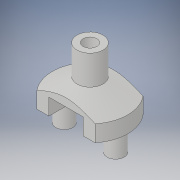
# Autodesk Inventor part: 1216.1001
Saved by Autodesk Inventor 2019.4 (Build 234330000, 330)
## iProperties
Created: 2019-11-11
Part Number: 1216.1001
Material: Generic
Document SubType Name: Modeling
Designer: phpgb
Density: 1 g/cm^3
Appearance: Default
Author: phpgb
Autodesk Inventor part; units mm, degrees
ref_plane "YZ Plane" through (0, 0, 0) normal (1, 0, 0) x (0, 1, 0)
ref_plane "XZ Plane" through (0, 0, 0) normal (0, 1, 0) x (-1, 0, 0)
ref_plane "XY Plane" through (0, 0, 0) normal (0, 0, 1) x (1, 0, 0)
sketch "Sketch1" plane through (0, 0, 0) normal (0, 1, 0) x (-1, 0, 0)
  line L0 (5.5, 3.5) -> (4.2426, 3.5) construction
  line L1 (-5.5, 3.5) -> (-5.5, -3.5) construction
  line L2 (-5.5, -3.5) -> (-4.2426, -3.5) construction
  line L3 (5.5, -3.5) -> (5.5, 3.5) construction
  line L4 (5.5, 3.5) -> (-5.5, -3.5) construction
  line L5 (-5.5, 3.5) -> (5.5, -3.5) construction
  arc A0 (4.2426, -3.5) -> (4.2426, 3.5) centre (0, 0) ccw
  line L6 (4.2426, -3.5) -> (5.5, -3.5) construction
  line L7 (-4.2426, -3.5) -> (4.2426, -3.5)
  line L8 (-4.2426, 3.5) -> (-5.5, 3.5) construction
  line L9 (4.2426, 3.5) -> (-4.2426, 3.5)
  arc A1 (-4.2426, -3.5) -> (4.2426, -3.5) centre (0, 0) ccw construction
  arc A2 (-4.2426, 3.5) -> (-4.2426, -3.5) centre (0, 0) ccw
  arc A3 (4.2426, 3.5) -> (-4.2426, 3.5) centre (0, 0) ccw construction
  circle A4 centre (0, 0) radius 1
  dimension "d0" = 11
  dimension "d1" = 7
  dimension "d2" = 11
  dimension "d3" = 2
  constraints: 20 end point, 10 parallel, 9 point on circle, 5 centre point, 3 horizontal, 3 perpendicular, 2 coincident, 2 midpoint
  measures "d0" distance of L3.start L1.end
  measures "d1" distance of L1.end L1.start
  measures "d2" diameter of A0
  measures "d3" diameter of A4
extrude "Extrusion1" add sketch "Sketch1" along normal blind 2.4
sketch "Sketch2" plane through (0, 0, 0) normal (0, -1, 0) x (1, 0, 0)
  circle A0 centre (0, 0) radius 1 construction
  arc A1 (-4.2426, 3.5) -> (-4.2426, -3.5) centre (0, 0) ccw construction
  line L0 (4.2426, -3.5) -> (-4.2426, -3.5) construction
  arc A2 (4.2426, -3.5) -> (4.2426, 3.5) centre (0, 0) ccw construction
  line L1 (-4.2426, 3.5) -> (4.2426, 3.5) construction
  arc A3 (-4.2426, 3.5) -> (-4.2426, -3.5) centre (0, 0) ccw construction
  line L2 (-5.5, 0) -> (5.5, 0) construction
  circle A4 centre (-3.75, 0) radius 1.25
  circle A5 centre (3.75, 0) radius 1.25
  line L3 (0, 3.5) -> (0, -3.5) construction
  circle A6 centre (-3.75, 0) radius 1.2
  circle A7 centre (3.75, 0) radius 1.2
  dimension "d6" = 2.5
  dimension "d7" = 2.5
  dimension "d8" = 7.5
  dimension "d9" = 3.75
  dimension "d10" = 2.4
  dimension "d11" = 2.4
  constraints: 4 centre point, 4 end point, 3 point on circle, 2 coincident, 2 midpoint, 2 point on line
  measures "d6" diameter of A4
  measures "d7" diameter of A5
  measures "d8" distance of A5.centre A4.centre
  measures "d9" distance from line of A4.centre L3
  measures "d10" diameter of A6
  measures "d11" diameter of A7
extrude "Extrusion2" add sketch "Sketch2" along normal blind 3.2 contours A4 | A5 | A6 | A7
sketch "Sketch3" plane through (0, 2.4, 0) normal (0, 1, 0) x (1, 0, 0)
  circle A0 centre (0, 0) radius 1.9
  circle A1 centre (0, 0) radius 1 projected
  dimension "d14" = 3.8
  constraints: 1 centre point, 1 coincident
  measures "d14" diameter of A0
extrude "Extrusion3" add sketch "Sketch3" along normal blind 6.4
chamfer "Chamfer1" distance 3.6 distance2 2.1 1 edges at (-1.9, 2.4, 0) measured on face at (-2.4, 2.4, 0)
sketch "Sketch5" plane through (-4.2426, 0, 3.5) normal (0, 0, 1) x (1, 0, 0)
  line L0 (1.7426, 0) -> (1.7426, -3.2) projected
  line L1 (1.7426, 0) -> (6.7426, 0)
  line L2 (6.7426, 0) -> (6.7426, 2.4)
  line L3 (6.7426, 2.4) -> (1.7426, 2.4)
  line L4 (1.7426, 2.4) -> (1.7426, 0)
  line L5 (0, 0) -> (8.4853, 0) projected
  line L6 (8.4853, 0) -> (8.4853, 2.4) projected
  line L7 (0, 0) -> (0, 2.4) projected
  point P0 (4.2426, 0)
  dimension "d22" = 5
  dimension "d23" = 2.4
  constraints: 8 end point, 2 parallel, 1 collinear, 1 horizontal, 1 horizontal alignment, 1 perpendicular, 1 point on line
  measures "d22" distance of L3.end L2.end
  measures "d23" distance of L2.end L1.end
extrude "Extrusion4" cut sketch "Sketch5" against normal up to surface (7 mm away)
equation "\"d9\" = 0.5 * d8"
body "Solid1"
